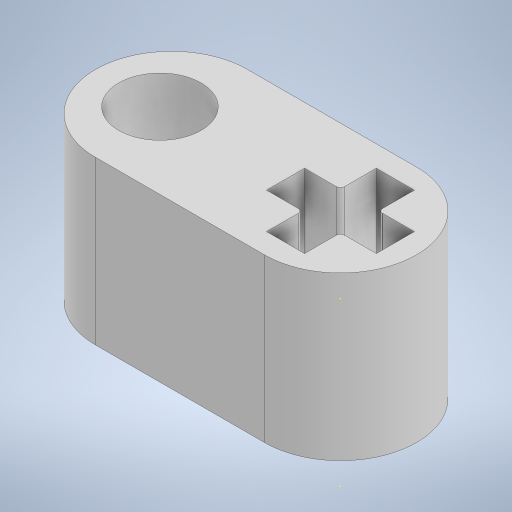
# Autodesk Inventor part: part1
Saved by Autodesk Inventor 2024 (Build 280153000, 153)
## iProperties
Created: 2023-10-06
Part Number: part1
Material: Generic
Document SubType Name: Modeling
Designer: kubad
Density: 1 g/cm^3
Appearance: Default
Author: kubad
## iProperties of the stored document part1_3DPrint.ipt
Created: 2023-10-06
Part Number: part1_3DPrint
Material: Generic
Document SubType Name: Modeling
Designer: kubad
Density: 1 g/cm^3
Appearance: Default
Author: kubad
Autodesk Inventor part; units mm, degrees
ref_plane "YZ Plane" through (0, 0, 0) normal (1, 0, 0) x (0, 1, 0)
ref_plane "XZ Plane" through (0, 0, 0) normal (0, 1, 0) x (-1, 0, 0)
ref_plane "XY Plane" through (0, 0, 0) normal (0, 0, 1) x (1, 0, 0)
sketch "Sketch1" plane through (0, 0, 0) normal (0, 1, 0) x (-1, 0, 0)
  point P0 (0, 0)
sketch "Sketch2" plane through (0, 0, 0) normal (0, 1, 0) x (-1, 0, 0)
  line L0 (0, 0) -> (15.2, 0)
  line L1 (15.2, 0) -> (15.2, -7.2)
  line L2 (15.2, -7.2) -> (0, -7.2)
  line L3 (0, -7.2) -> (0, 0)
  dimension "d0" = 15.2
  dimension "d1" = 7.2
  constraints: 8 end point, 2 parallel, 1 horizontal, 1 perpendicular
  measures "d0" distance of L1.end L2.end
  measures "d1" distance of L0.end L1.end
extrude "Extrusion1" add sketch "Sketch2" along normal blind 7.7
fillet "Fillet1" radius 3.6 2 edges at (0, 3.85, 0) (0, 3.85, -7.2)
fillet "Fillet2" radius 3.6 2 edges at (-15.2, 3.85, 0) (-15.2, 3.85, -7.2)
sketch "Sketch3" plane through (0, 7.7, 0) normal (0, 1, 0) x (1, 0, 0)
  arc A0 (-3.6, 0) -> (-3.6, 7.2) centre (-3.6, 3.6) ccw projected
  line L0 (0, 3.6) -> (-1, 3.6)
  line L1 (-1, 3.6) -> (-1, 4.5)
  line L2 (-1, 3.6) -> (-1, 2.7)
  line L3 (-1, 4.5) -> (-5.8, 4.5)
  line L4 (-5.8, 4.5) -> (-5.8, 2.7)
  line L5 (-5.8, 2.7) -> (-1, 2.7)
  line L6 (-1, 2.7) -> (-1, 4.5)
  line L7 (-1, 3.6) -> (-3.4, 3.6)
  line L8 (-3.4, 3.6) -> (-3.4, 6)
  line L9 (-3.4, 3.6) -> (-3.4, 1.2)
  line L10 (-3.4, 6) -> (-2.5, 6)
  line L11 (-3.4, 6) -> (-4.3, 6)
  line L12 (-4.3, 6) -> (-2.5, 6)
  line L13 (-2.5, 6) -> (-2.5, 1.2)
  line L14 (-2.5, 1.2) -> (-4.3, 1.2)
  line L15 (-4.3, 1.2) -> (-4.3, 6)
  point P0 (0, 0)
  point P1 (-4.3, 2.7)
  point P2 (-4.3, 4.5)
  point P3 (-2.5, 4.5)
  point P4 (-3.4, 4.5)
  point P5 (-2.5, 2.7)
  point P6 (-3.4, 2.7)
  dimension "d6" = 1
  dimension "d14" = 0.9
  dimension "d15" = 0.9
  dimension "d16" = 4.8
  dimension "d17" = 2.4
  dimension "d18" = 2.4
  dimension "d19" = 0.9
  dimension "d20" = 0.9
  dimension "d21" = 4.8
  constraints: 32 end point, 5 horizontal, 4 parallel, 4 vertical, 2 perpendicular, 1 point on circle
  measures "d6" distance of L0.start L0.end
  measures "d14" distance of L0.end L1.end
  measures "d15" distance of L0.end L2.end
  measures "d16" distance of L5.end L4.end
  measures "d17" distance of L7.end L8.end
  measures "d18" distance of L7.end L9.end
  measures "d19" distance of L8.end L10.end
  measures "d20" distance of L8.end L11.end
  measures "d21" distance of L12.end L13.end
extrude "Extrusion2" cut sketch "Sketch3" against normal through all contours L15 L5 L4 L3
extrude "Extrusion3" cut sketch "Sketch3" against normal through all contours L3 L8 L10 L13
extrude "Extrusion4" cut sketch "Sketch3" against normal through all contours L3 L15 L11 L8
extrude "Extrusion5" cut sketch "Sketch3" against normal through all contours L13 L14 L9 L5
extrude "Extrusion6" cut sketch "Sketch3" against normal through all contours L9 L14 L15 L5
extrude "Extrusion7" cut sketch "Sketch3" against normal through all contours L7 L13 L3 L1 | L2 L5 L13 L7 | L13 L5 L9 L7 | L7 L8 L3 L13 | L9 L5 L15 L3 L8 | L15 L5 L4 L3
fillet "Fillet3" radius 0.2 1 edges at (-4.3, 3.85, -4.5)
fillet "Fillet4" radius 0.2 1 edges at (-4.3, 3.85, -2.7)
fillet "Fillet5" radius 0.2 1 edges at (-2.5, 3.85, -2.7)
fillet "Fillet6" radius 0.2 1 edges at (-2.5, 3.85, -4.5)
sketch "Sketch4" plane through (0, 7.7, 0) normal (0, 1, 0) x (1, 0, 0)
  arc A0 (-11.6, 7.2) -> (-11.6, 0) centre (-11.6, 3.6) ccw projected
  line L0 (-15.2, 3.6) -> (-14, 3.6)
  line L1 (-14, 3.6) -> (-10.3, 3.6)
  circle A1 centre (-12.15, 3.6) radius 1.85
  point P0 (0, 0)
  dimension "d38" = 1.2
  dimension "d39" = 3.7
  constraints: 4 end point, 2 horizontal, 1 horizontal alignment, 1 midpoint, 1 point on circle, 2 other
  measures "d38" distance of L0.start L0.end
  measures "d39" distance of L0.end L1.end
extrude "Extrusion8" cut sketch "Sketch4" against normal through all
sketch "Sketch5" plane through (-3.6, 0, 0) normal (0, 0, 1) x (1, 0, 0)
  line L0 (-6.2992, 6.9034) -> (0.3672, 6.9034) construction
  line L1 (0.3672, 6.9034) -> (0.3672, 0.2653) construction
  line L2 (0.3672, 0.2653) -> (-6.2992, 0.2653) construction
  line L3 (-6.2992, 0.2653) -> (-6.2992, 6.9034) construction
  spline S0 degree 2 poles (-1.5438, 2.6769) (-1.5438, 2.2221) (-1.8898, 1.5251) (-2.1766, 1.2977) knots 0 0 0 1 2 2 2
  spline S1 degree 2 poles (-2.1766, 1.2977) (-2.5226, 1.0308) (-3.3086, 0.8034) (-3.9314, 0.8034) knots 0 0 0 1 2 2 2
  line L4 (-3.9314, 0.8034) -> (-5.6813, 0.8034)
  line L5 (-5.6813, 0.8034) -> (-5.6813, 6.9034)
  line L6 (-5.6813, 6.9034) -> (-4.0649, 6.9034)
  spline S2 degree 2 poles (-4.0649, 6.9034) (-3.4124, 6.9034) (-2.7599, 6.8193) (-2.4633, 6.6562) knots 0 0 0 1 2 2 2
  spline S3 degree 2 poles (-2.4633, 6.6562) (-2.1321, 6.4832) (-1.8305, 5.9147) (-1.8305, 5.5292) knots 0 0 0 1 2 2 2
  spline S4 degree 2 poles (-1.8305, 5.5292) (-1.8305, 5.0991) (-2.2853, 4.4169) (-2.6857, 4.2241) knots 0 0 0 1 2 2 2
  line L7 (-2.6857, 4.2241) -> (-2.6857, 4.1945)
  spline S5 degree 2 poles (-2.6857, 4.1945) (-2.142, 4.0462) (-1.5438, 3.2602) (-1.5438, 2.6769) knots 0 0 0 1 2 2 2
  spline S6 degree 2 poles (-2.3891, 2.6423) (-2.3891, 2.9883) (-2.5868, 3.4332) (-2.8834, 3.5914) knots 0 0 0 1 2 2 2
  spline S7 degree 2 poles (-2.8834, 3.5914) (-3.0762, 3.6903) (-3.531, 3.7496) (-3.9512, 3.7496) knots 0 0 0 1 2 2 2
  line L8 (-3.9512, 3.7496) -> (-4.8706, 3.7496)
  line L9 (-4.8706, 3.7496) -> (-4.8706, 1.4954)
  line L10 (-4.8706, 1.4954) -> (-4.2132, 1.4954)
  spline S8 degree 2 poles (-4.2132, 1.4954) (-3.6793, 1.4954) (-3.0663, 1.5943) (-2.8291, 1.7525) knots 0 0 0 1 2 2 2
  spline S9 degree 2 poles (-2.8291, 1.7525) (-2.6017, 1.9156) (-2.3891, 2.321) (-2.3891, 2.6423) knots 0 0 0 1 2 2 2
  spline S10 degree 2 poles (-2.6758, 5.4155) (-2.6758, 5.633) (-2.8241, 5.9592) (-2.9873, 6.0531) knots 0 0 0 1 2 2 2
  spline S11 degree 2 poles (-2.9873, 6.0531) (-3.185, 6.1619) (-3.6645, 6.2113) (-4.0945, 6.2113) knots 0 0 0 1 2 2 2
  line L11 (-4.0945, 6.2113) -> (-4.8706, 6.2113)
  line L12 (-4.8706, 6.2113) -> (-4.8706, 4.4268)
  line L13 (-4.8706, 4.4268) -> (-3.9512, 4.4268)
  spline S12 degree 2 poles (-3.9512, 4.4268) (-3.5706, 4.4268) (-3.2097, 4.5059) (-3.0169, 4.6295) knots 0 0 0 1 2 2 2
  spline S13 degree 2 poles (-3.0169, 4.6295) (-2.8291, 4.7481) (-2.6758, 5.1287) (-2.6758, 5.4155) knots 0 0 0 1 2 2 2
  point P0 (3.6, 0)
  constraints: 2 other
extrude "Extrusion9" cut sketch "Sketch5" against normal blind 0.2
sketch "Sketch6" plane through (0, 7.7, 0) normal (0, 1, 0) x (1, 0, 0)
  circle A0 centre (-12.15, 3.6) radius 1.85 projected
  circle A1 centre (-12.15, 3.6) radius 1.95
  point P0 (0, 0)
  dimension "d44" = 3.9
  constraints: 1 centre point, 1 coincident
  measures "d44" diameter of A1
extrude "Extrusion10" cut sketch "Sketch6" against normal through all
sketch "Sketch7" plane through (0, 7.7, 0) normal (0, 1, 0) x (1, 0, 0)
  line L0 (-4.3, 4.5) -> (-4.7532, 4.5)
  line L1 (-4.7532, 4.5) -> (-4.7532, 4.9695)
  line L2 (-4.7532, 4.9695) -> (-4.3, 4.9695)
  line L3 (-4.3, 4.9695) -> (-4.3, 4.5)
  arc A0 (-2.5, 4.7) -> (-2.3, 4.5) centre (-2.3, 4.7) ccw projected
  line L4 (-2.3, 4.7) -> (-2.5, 4.7)
  line L5 (-2.5, 4.7) -> (-2.5, 4.5)
  line L6 (-2.5, 4.5) -> (-2.3, 4.5)
  line L7 (-2.3, 4.5) -> (-2.3, 4.7)
  arc A1 (-2.3, 2.7) -> (-2.5, 2.5) centre (-2.3, 2.5) ccw projected
  line L8 (-2.3, 2.5) -> (-2.5, 2.5)
  line L9 (-2.5, 2.5) -> (-2.5, 2.7)
  line L10 (-2.5, 2.7) -> (-2.3, 2.7)
  line L11 (-2.3, 2.7) -> (-2.3, 2.5)
  arc A2 (-4.3, 2.5) -> (-4.5, 2.7) centre (-4.5, 2.5) ccw projected
  line L12 (-4.5, 2.5) -> (-4.3, 2.5)
  line L13 (-4.3, 2.5) -> (-4.3, 2.7)
  line L14 (-4.3, 2.7) -> (-4.5, 2.7)
  line L15 (-4.5, 2.7) -> (-4.5, 2.5)
  point P0 (0, 0)
  constraints: 32 end point, 8 parallel, 4 horizontal, 4 perpendicular, 1 point on line
extrude "Extrusion11" add sketch "Sketch7" against normal blind 7.7 contours L0 L1 L2 L3
extrude "Extrusion12" add sketch "Sketch7" against normal blind 7.7 contours L4 L7 A0 | A0 L6 L5
extrude "Extrusion13" add sketch "Sketch7" against normal blind 7.7 contours L12 L15 A2 | A2 L14 L13
extrude "Extrusion14" add sketch "Sketch7" against normal blind 7.7 contours L11 L8 A1 | A1 L9 L10
sketch "Sketch8" plane through (0, 7.7, 0) normal (0, 1, 0) x (1, 0, 0)
  line L0 (-2.5, 2.7) -> (-1, 2.7) projected
  line L1 (-4.3, 1.2) -> (-2.5, 1.2) projected
  line L2 (-2.5, 2.7) -> (-2.7, 2.7)
  line L3 (-2.7, 2.7) -> (-2.7, 1.2)
  line L4 (-2.7, 1.2) -> (-2.5, 1.2)
  line L5 (-2.5, 1.2) -> (-2.5, 2.7)
  line L6 (-2.5, 6) -> (-4.3, 6) projected
  line L7 (-2.5, 6) -> (-2.7, 6)
  line L8 (-2.7, 6) -> (-2.7, 4.4977)
  line L9 (-2.7, 4.4977) -> (-2.5, 4.4977)
  line L10 (-2.5, 4.4977) -> (-2.5, 6)
  line L11 (-4.3, 4.5) -> (-5.8, 4.5) projected
  line L12 (-5.8, 4.5) -> (-6, 4.5)
  line L13 (-6, 4.5) -> (-6, 2.7)
  line L14 (-6, 2.7) -> (-5.8, 2.7)
  line L15 (-5.8, 2.7) -> (-5.8, 4.5)
  line L16 (-4.3, 6) -> (-4.5, 6)
  line L17 (-4.5, 6) -> (-4.5, 4.5)
  line L18 (-4.5, 4.5) -> (-4.3, 4.5)
  line L19 (-4.3, 4.5) -> (-4.3, 6)
  line L20 (-4.3, 2.7) -> (-4.3, 1.2) projected
  line L21 (-4.3, 2.7) -> (-4.5, 2.7)
  line L22 (-4.5, 2.7) -> (-4.5, 1.2)
  line L23 (-4.5, 1.2) -> (-4.3, 1.2)
  line L24 (-4.3, 1.2) -> (-4.3, 2.7)
  point P0 (0, 0)
  dimension "d55" = 0.2
  dimension "d56" = 0.2
  dimension "d57" = 0.2
  dimension "d58" = 0.2
  dimension "d59" = 0.2
  constraints: 40 end point, 10 parallel, 5 horizontal, 5 perpendicular, 2 point on line
  measures "d55" distance of L4.end L3.end
  measures "d56" distance of L9.end L8.end
  measures "d57" distance of L14.end L13.end
  measures "d58" distance of L18.end L17.end
  measures "d59" distance of L23.end L22.end
extrude "Extrusion15" add sketch "Sketch8" against normal blind 7.7 contours L10 L9 L8 L6
extrude "Extrusion16" add sketch "Sketch8" against normal blind 7.7 contours L3 L2 L5 L1
extrude "Extrusion17" cut sketch "Sketch8" against normal through all contours L19 L11 L17 L16
extrude "Extrusion18" cut sketch "Sketch8" against normal through all contours L23 L22 L21 L20
extrude "Extrusion19" cut sketch "Sketch8" against normal through all contours L15 L14 L13 L12
sketch "Sketch9" plane through (0, 7.7, 0) normal (0, 1, 0) x (1, 0, 0)
  point P0 (0, 0)
sketch "Sketch10" plane through (0, 7.7, 0) normal (0, 1, 0) x (1, 0, 0)
  line L0 (-6, 4.5) -> (-4.5, 4.5) projected
  line L1 (-2.7, 2.7) -> (-2.7, 1.2) projected
  line L2 (-4.5, 4.5) -> (-2.7, 4.5)
  line L3 (-2.7, 4.5) -> (-2.7, 2.7)
  line L4 (-2.7, 2.7) -> (-4.5, 2.7)
  line L5 (-4.5, 2.7) -> (-4.5, 4.5)
  line L6 (-4.5, 6) -> (-2.7, 6) projected
  line L7 (-4.5, 6) -> (-2.7, 6)
  line L8 (-2.7, 6) -> (-2.7, 6.2)
  line L9 (-2.7, 6.2) -> (-4.5, 6.2)
  line L10 (-4.5, 6.2) -> (-4.5, 6)
  line L11 (-6, 4.5) -> (-6.2, 4.5)
  line L12 (-6.2, 4.5) -> (-6.2, 2.7)
  line L13 (-6.2, 2.7) -> (-6, 2.7)
  line L14 (-6, 2.7) -> (-6, 4.5)
  line L15 (-2.7, 1.2) -> (-4.5, 1.2)
  line L16 (-4.5, 1.2) -> (-4.5, 1)
  line L17 (-4.5, 1) -> (-2.7, 1)
  line L18 (-2.7, 1) -> (-2.7, 1.2)
  point P0 (0, 0)
  dimension "d70" = 0.2
  dimension "d71" = 0.2
  dimension "d72" = 0.2
  constraints: 32 end point, 8 parallel, 4 horizontal, 4 perpendicular
  measures "d70" distance of L8.end L7.end
  measures "d71" distance of L13.end L12.end
  measures "d72" distance of L16.end L15.end
extrude "Extrusion20" cut sketch "Sketch10" against normal through all contours L10 L9 L8 L6
extrude "Extrusion21" cut sketch "Sketch10" against normal through all contours L14 L13 L12 L11
extrude "Extrusion22" cut sketch "Sketch10" against normal through all contours L18 L17 L16 L15
fillet "Fillet7" radius 0.2 1 edges at (-4.5, 3.85, -4.5)
fillet "Fillet8" radius 0.2 1 edges at (-2.7, 3.85, -4.4977)
fillet "Fillet9" radius 0.2 1 edges at (-2.7, 3.85, -2.7)
fillet "Fillet10" radius 0.2 1 edges at (-4.5, 3.85, -2.7)
sketch "Sketch11" plane through (-3.6, 0, 0) normal (0, 0, 1) x (1, 0, 0)
  line L0 (-7.3139, 7.2702) -> (-0.5941, 7.2702)
  line L1 (-0.5941, 7.2702) -> (-0.5941, 0.3916)
  line L2 (-0.5941, 0.3916) -> (-7.3139, 0.3916)
  line L3 (-7.3139, 0.3916) -> (-7.3139, 7.2702)
  point P0 (3.6, 0)
  constraints: 8 end point, 2 parallel, 1 horizontal, 1 perpendicular
extrude "Extrusion23" add sketch "Sketch11" against normal blind 0.5
body "Solid1"
